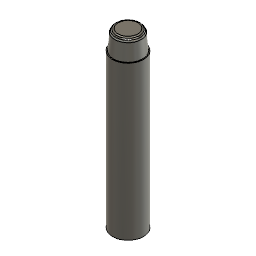
Dart (Autodesk Fusion 360 design; units mm, degrees)
part number: 2026-08-22-19-50-19-504
Autodesk Fusion 360 part; units mm, degrees
cylinder "CylinderPrimitive2" add diameter 13 height 64 placed x (1, 0, 0) y (0, 0, -1) z (0, 1, 0) at (0, 0, 0)
sketch "Sketch6" plane through (0, 64, 0) normal (0, 1, 0) x (-1, 0, 0)
  circle A0 centre (0, 0) radius 6.5
  circle A1 centre (0, 0) radius 6.1
  dimension "d16" = 12.2
  constraint coincident A0.centre A1.centre
  measures "d16" diameter of A1
ref_plane "WorkPlane2" through (0, 72, 0) normal (0, 1, 0) x (-1, 0, 0)
ref_plane "WorkPlane3" through (0, 71.087, 0) normal (0, 1, 0) x (-1, 0, 0)
sketch "Sketch7" plane through (0, 71.087, 0) normal (0, 1, 0) x (1, 0, 0)
  circle A0 centre (0, 0) radius 5.48
  dimension "d21" = 10.96
  constraint coincident A0.centre origin
  measures "d21" diameter of A0
sketch "Sketch8" plane through (0, 72, 0) normal (0, 1, 0) x (1, 0, 0)
  circle A0 centre (0, 0) radius 4.484
  dimension "d22" = 8.968
  constraint coincident A0.centre origin
  measures "d22" diameter of A0
loft "Loft2" add profiles "Sketch6", "Sketch7" section 1 contours A1 section 2
loft "Loft3" add profiles "Sketch8" section 1 face at (-0.7564, 71.087, -0.0326) section 2
fillet "Fillet2" radius 1 1 faces at (-5.1416, 71.3913, -0.2566)
